Autodesk Fusion 360 part; units mm, degrees
(part 2 of 5)
  spline S130 degree 3 poles (60.3737, -55.5609) (60.3438, -55.5896) (60.2486, -55.657) (60.1179, -55.7383) (59.8305, -55.9172) (59.3718, -56.1632) (59.06, -56.2112) knots 43 43 43 43 44 44 44 45 45 45 45
  spline S131 degree 3 poles (59.06, -56.2112) (58.9588, -56.2268) (58.9104, -56.219) (58.892, -56.2135) knots 45 45 45 45 46 46 46 46
  spline S132 degree 3 poles (58.892, -56.2135) (58.8899, -56.1496) (58.9675, -55.9719) (59.1151, -55.7925) knots 46 46 46 46 47 47 47 47
  ellipse E15 centre (57.3205, -53.9765) end of major axis (56.0356, -51.7283) minor radius 2.1626 (59.1151, -55.7925) -> (59.5802, -54.6452) ccw
  ellipse E16 centre (59.4059, -54.626) end of major axis (59.3998, -54.4501) minor radius 0.1753 (59.5802, -54.6452) -> (59.5256, -54.4974) ccw
  ellipse E17 centre (59.4023, -54.6266) end of major axis (59.2635, -54.7391) minor radius 0.1761 (59.5256, -54.4974) -> (59.3747, -54.4521) ccw
  spline S133 degree 3 poles (59.3747, -54.4521) (55.9933, -55.04) (49.7205, -55.3474) (45.6899, -50.8019) knots 50 50 50 50 51 51 51 51
  ellipse E18 centre (53.6278, -44.8754) end of major axis (44.2457, -38.0609) minor radius 9.7795 (43.9053, -48.2176) -> (45.6899, -50.8019) ccw
  line L25 (43.9053, -48.2176) -> (43.8433, -48.0971)
  ellipse E19 centre (49.3851, -44.1794) end of major axis (52.1384, -53.1388) minor radius 6.6191 (42.9149, -45.6233) -> (43.8433, -48.0971) ccw
  ellipse E20 centre (51.6421, -43.1384) end of major axis (52.985, -53.2351) minor radius 9.0542 (42.8875, -40.1596) -> (42.9149, -45.6233) ccw
  arc A2 (42.8875, -40.1596) -> (42.9826, -39.7986) centre (53.3142, -42.7132) cw
  ellipse E21 centre (42.8151, -39.7494) end of major axis (42.7434, -39.5895) minor radius 0.1739 (42.9826, -39.7986) -> (42.9638, -39.6591) ccw
  spline S134 degree 3 poles (42.9638, -39.6591) (42.3811, -38.6984) (41.6291, -37.8042) (40.8669, -37.0262) (39.8868, -36.026) (38.8897, -35.2179) (38.2132, -34.708) (37.6172, -34.2587) (37.2267, -34.0054) (37.2179, -34.0001) knots 57 57 57 57 58 58 58 59 59 59 60 60 60 60
  ellipse E22 centre (35.2958, -35.3818) end of major axis (31.3426, -33.1165) minor radius 2.2062 (37.2179, -34.0001) -> (36.1564, -33.3367) ccw
  spline S135 degree 3 poles (36.1564, -33.3367) (36.076, -33.2937) (35.9763, -33.3192) (35.9263, -33.3948) knots 61 61 61 61 62 62 62 62
  line L26 (35.9263, -33.3948) -> (35.5901, -33.9003)
  spline S136 degree 3 poles (35.5901, -33.9003) (34.94, -34.8769) (34.2677, -35.8869) (33.6646, -36.9182) knots 63 63 63 63 64 64 64 64
  spline S137 degree 3 poles (33.6646, -36.9182) (33.2824, -37.5723) (32.9384, -38.2578) (32.6058, -38.9206) knots 64 64 64 64 65 65 65 65
  spline S138 degree 3 poles (32.6058, -38.9206) (32.2773, -39.5755) (31.9376, -40.2527) (31.5629, -40.8949) (31.5163, -40.9748) (31.47, -41.0529) (31.4239, -41.1294) knots 65 65 65 65 66 66 66 67 67 67 67
  spline S139 degree 3 poles (31.4239, -41.1294) (31.1015, -41.6648) (30.7918, -42.1186) (30.481, -42.5114) knots 67 67 67 67 68 68 68 68
  line L27 (30.481, -42.5114) -> (30.4362, -42.5696)
  spline S140 degree 3 poles (30.4362, -42.5696) (30.4117, -42.6016) (30.3873, -42.6336) (30.362, -42.6641) knots 69 69 69 69 70 70 70 70
  spline S141 degree 3 poles (30.362, -42.6641) (30.3582, -42.6686) (30.3547, -42.6734) (30.3515, -42.6783) knots 70 70 70 70 71 71 71 71
  spline S142 degree 3 poles (30.3515, -42.6783) (30.3203, -42.7234) (28.6461, -45.1229) (26.2909, -45.4412) knots 71 71 71 71 72 72 72 72
  ellipse E23 centre (26.3128, -35.2005) end of major axis (25.464, -45.4631) minor radius 6.2326 (24.6688, -45.3108) -> (26.2909, -45.4412) ccw
  spline S143 degree 3 poles (24.6688, -45.3108) (24.6431, -45.2963) (24.618, -45.2804) (24.5928, -45.2647) knots 73 73 73 73 74 74 74 74
  line L28 (24.5928, -45.2647) -> (24.5503, -45.2383)
  spline S144 degree 3 poles (24.5503, -45.2383) (24.3504, -45.1156) (24.1596, -44.9484) (23.9667, -44.7273) knots 75 75 75 75 76 76 76 76
  spline S145 degree 3 poles (23.9667, -44.7273) (23.8509, -44.594) (23.7755, -44.4771) (23.7295, -44.3593) knots 76 76 76 76 77 77 77 77
  ellipse E24 centre (23.8379, -44.243) end of major axis (24.0045, -44.7223) minor radius 0.1422 (23.6258, -43.858) -> (23.7295, -44.3593) ccw
  ellipse E25 centre (25.0663, -43.2544) end of major axis (23.7372, -44.3058) minor radius 0.9128 (23.7072, -43.5372) -> (23.6258, -43.858) ccw
  ellipse E26 centre (23.7572, -43.5067) end of major axis (23.6649, -43.7209) minor radius 0.0345 (23.7632, -43.412) -> (23.7072, -43.5372) ccw
  spline S146 degree 3 poles (23.7632, -43.412) (23.9002, -43.2702) (24.0362, -43.1231) (24.1722, -42.9764) knots 80 80 80 80 81 81 81 81
  line L29 (24.1722, -42.9764) -> (24.3262, -42.8105)
  ellipse E27 centre (22.2632, -42.3236) end of major axis (19.1066, -44.8285) minor radius 1.7599 (24.3262, -42.8105) -> (24.9513, -42.0428) ccw
  spline S147 degree 3 poles (24.9513, -42.0428) (25.0276, -41.933) (25.103, -41.8145) (25.1819, -41.6801) knots 83 83 83 83 84 84 84 84
  spline S148 degree 3 poles (25.1819, -41.6801) (25.1991, -41.6508) (25.215, -41.6211) (25.231, -41.5914) knots 84 84 84 84 85 85 85 85
  line L30 (25.231, -41.5914) -> (25.2527, -41.5513)
  spline S149 degree 3 poles (25.2527, -41.5513) (25.2973, -41.4707) (25.3416, -41.3895) (25.3826, -41.3066) knots 86 86 86 86 87 87 87 87
  spline S150 degree 3 poles (25.3826, -41.3066) (25.4022, -41.2663) (25.4208, -41.2258) (25.4396, -41.1853) knots 87 87 87 87 88 88 88 88
  line L31 (25.4396, -41.1853) -> (25.4579, -41.1455)
  spline S151 degree 3 poles (25.4579, -41.1455) (25.4913, -41.0727) (25.5238, -40.9995) (25.5543, -40.9255) (25.5791, -40.8653) (25.6029, -40.8046) (25.626, -40.7437) knots 89 89 89 89 90 90 90 91 91 91 91
  spline S152 degree 3 poles (25.626, -40.7437) (25.6517, -40.6761) (25.6761, -40.6074) (25.6997, -40.5385) knots 91 91 91 91 92 92 92 92
  spline S153 degree 3 poles (25.6997, -40.5385) (25.7223, -40.4724) (25.7448, -40.4057) (25.7657, -40.3384) knots 92 92 92 92 93 93 93 93
  spline S154 degree 3 poles (25.7657, -40.3384) (25.7846, -40.277) (25.802, -40.2143) (25.8187, -40.1532) knots 93 93 93 93 94 94 94 94
  line L32 (25.8187, -40.1532) -> (25.8311, -40.1093)
  spline S155 degree 3 poles (25.8311, -40.1093) (25.848, -40.0494) (25.8649, -39.9896) (25.8804, -39.9277) knots 95 95 95 95 96 96 96 96
  line L33 (25.8804, -39.9277) -> (25.9066, -39.8117)
  spline S156 degree 3 poles (25.9066, -39.8117) (25.9578, -39.5907) (26, -39.3731) (26.0332, -39.1571) (26.1059, -38.6843) (26.1474, -38.1845) (26.1602, -37.6287) knots 97 97 97 97 98 98 98 99 99 99 99
  line L34 (26.1602, -37.6287) -> (26.1614, -37.5503)
  spline S157 degree 3 poles (26.1614, -37.5503) (26.1634, -37.4115) (26.1648, -37.2726) (26.1634, -37.1358) knots 100 100 100 100 101 101 101 101
  line L35 (26.1634, -37.1358) -> (26.1622, -37.0204)
  spline S158 degree 3 poles (26.1622, -37.0204) (26.1607, -36.8934) (26.1581, -36.7667) (26.1539, -36.6415) knots 102 102 102 102 103 103 103 103
  line L36 (26.1539, -36.6415) -> (26.1496, -36.5105)
  spline S159 degree 3 poles (26.1496, -36.5105) (26.145, -36.3889) (26.1397, -36.2682) (26.1333, -36.1463) knots 104 104 104 104 105 105 105 105
  line L37 (26.1333, -36.1463) -> (26.1266, -36.0149)
  spline S160 degree 3 poles (26.1266, -36.0149) (26.1195, -35.8921) (26.1119, -35.7703) (26.1037, -35.6507) knots 106 106 106 106 107 107 107 107
  line L38 (26.1037, -35.6507) -> (26.0961, -35.5324)
  spline S161 degree 3 poles (26.0961, -35.5324) (26.0852, -35.376) (26.0738, -35.2208) (26.0618, -35.0674) (26.0421, -34.8173) (26.0218, -34.5675) (26.0015, -34.3178) (25.98, -34.0538) (25.9584, -33.7898) (25.9378, -33.5252) knots 108 108 108 108 109 109 109 110 110 110 111 111 111 111
  spline S162 degree 3 poles (25.9378, -33.5252) (25.9371, -33.5162) (25.9357, -33.5074) (25.9336, -33.4988) knots 111 111 111 111 112 112 112 112
  line L39 (25.9336, -33.4988) -> (25.9306, -33.464)
  spline S163 degree 3 poles (25.9306, -33.464) (25.9294, -33.4503) (25.9283, -33.4366) (25.927, -33.4216) knots 113 113 113 113 114 114 114 114
  spline S164 degree 3 poles (25.927, -33.4216) (25.925, -33.3993) (25.9229, -33.3745) (25.9208, -33.3495) knots 114 114 114 114 115 115 115 115
  spline S165 degree 3 poles (25.9208, -33.3495) (25.9196, -33.3359) (25.9185, -33.3227) (25.9172, -33.3084) knots 115 115 115 115 116 116 116 116
  spline S166 degree 3 poles (25.9172, -33.3084) (25.9146, -33.2781) (25.9119, -33.2454) (25.909, -33.2118) (25.9081, -33.2012) (25.9073, -33.191) (25.9063, -33.18) knots 116 116 116 116 117 117 117 118 118 118 118
  spline S167 degree 3 poles (25.9063, -33.18) (25.9034, -33.1453) (25.9003, -33.1082) (25.8971, -33.0705) knots 118 118 118 118 119 119 119 119
  spline S168 degree 3 poles (25.8971, -33.0705) (25.896, -33.0568) (25.8949, -33.0437) (25.8937, -33.0296) knots 119 119 119 119 120 120 120 120
  spline S169 degree 3 poles (25.8937, -33.0296) (25.8907, -32.994) (25.8876, -32.9561) (25.8844, -32.9181) knots 120 120 120 120 121 121 121 121
  spline S170 degree 3 poles (25.8844, -32.9181) (25.8827, -32.8984) (25.8812, -32.8793) (25.8795, -32.859) knots 121 121 121 121 122 122 122 122
  spline S171 degree 3 poles (25.8795, -32.859) (25.8768, -32.8266) (25.874, -32.7925) (25.8712, -32.7586) knots 122 122 122 122 123 123 123 123
  line L40 (25.8712, -32.7586) -> (25.8643, -32.6743)
  spline S172 degree 3 poles (25.8643, -32.6743) (25.8616, -32.6416) (25.8589, -32.6075) (25.8561, -32.5735) knots 124 124 124 124 125 125 125 125
  spline S173 degree 3 poles (25.8561, -32.5735) (25.8538, -32.5439) (25.8514, -32.5146) (25.8489, -32.4841) knots 125 125 125 125 126 126 126 126
  spline S174 degree 3 poles (25.8489, -32.4841) (25.8459, -32.4468) (25.8428, -32.408) (25.8398, -32.3695) knots 126 126 126 126 127 127 127 127
  spline S175 degree 3 poles (25.8398, -32.3695) (25.8373, -32.3384) (25.8348, -32.3078) (25.8323, -32.276) knots 127 127 127 127 128 128 128 128
  spline S176 degree 3 poles (25.8323, -32.276) (25.8295, -32.2409) (25.8267, -32.2044) (25.8238, -32.1684) knots 128 128 128 128 129 129 129 129
  spline S177 degree 3 poles (25.8238, -32.1684) (25.8209, -32.1317) (25.8181, -32.0952) (25.8151, -32.0577) knots 129 129 129 129 130 130 130 130
  spline S178 degree 3 poles (25.8151, -32.0577) (25.812, -32.0184) (25.8089, -31.978) (25.8058, -31.9378) knots 130 130 130 130 131 131 131 131
  spline S179 degree 3 poles (25.8058, -31.9378) (25.8032, -31.9041) (25.8006, -31.8707) (25.798, -31.8364) knots 131 131 131 131 132 132 132 132
  spline S180 degree 3 poles (25.798, -31.8364) (25.794, -31.7852) (25.7901, -31.7329) (25.7861, -31.6805) knots 132 132 132 132 133 133 133 133
  spline S181 degree 3 poles (25.7861, -31.6805) (25.7842, -31.656) (25.7824, -31.6318) (25.7805, -31.6069) knots 133 133 133 133 134 134 134 134
  spline S182 degree 3 poles (25.7805, -31.6069) (25.7765, -31.5529) (25.7724, -31.4979) (25.7683, -31.4428) knots 134 134 134 134 135 135 135 135
  spline S183 degree 3 poles (25.7683, -31.4428) (25.7663, -31.4157) (25.7643, -31.3889) (25.7622, -31.3615) knots 135 135 135 135 136 136 136 136
  spline S184 degree 3 poles (25.7622, -31.3615) (25.7584, -31.3084) (25.7544, -31.2545) (25.7505, -31.2006) knots 136 136 136 136 137 137 137 137
  spline S185 degree 3 poles (25.7505, -31.2006) (25.7484, -31.1715) (25.7463, -31.1426) (25.7442, -31.1133) (25.7405, -31.0623) (25.7368, -31.0107) (25.7332, -30.9591) knots 137 137 137 137 138 138 138 139 139 139 139
  spline S186 degree 3 poles (25.7332, -30.9591) (25.7307, -30.9247) (25.7283, -30.8905) (25.7259, -30.8558) knots 139 139 139 139 140 140 140 140
  spline S187 degree 3 poles (25.7259, -30.8558) (25.722, -30.8009) (25.7182, -30.7456) (25.7144, -30.6902) (25.7124, -30.6617) (25.7104, -30.6333) (25.7085, -30.6046) knots 140 140 140 140 141 141 141 142 142 142 142
  spline S188 degree 3 poles (25.7085, -30.6046) (25.7045, -30.5466) (25.7006, -30.4883) (25.6967, -30.4299) knots 142 142 142 142 143 143 143 143
  spline S189 degree 3 poles (25.6967, -30.4299) (25.6948, -30.4007) (25.6928, -30.3716) (25.6908, -30.3424) (25.6869, -30.2824) (25.683, -30.2223) (25.6791, -30.1622) knots 143 143 143 143 144 144 144 145 145 145 145
  spline S190 degree 3 poles (25.6791, -30.1622) (25.6775, -30.136) (25.6758, -30.11) (25.6741, -30.0838) knots 145 145 145 145 146 146 146 146
  spline S191 degree 3 poles (25.6741, -30.0838) (25.6703, -30.0249) (25.6667, -29.966) (25.663, -29.9072) knots 146 146 146 146 147 147 147 147
  spline S192 degree 3 poles (25.663, -29.9072) (25.6613, -29.878) (25.6594, -29.8489) (25.6576, -29.8198) knots 147 147 147 147 148 148 148 148
  spline S193 degree 3 poles (25.6576, -29.8198) (25.6543, -29.766) (25.6512, -29.7126) (25.648, -29.659) knots 148 148 148 148 149 149 149 149
  spline S194 degree 3 poles (25.648, -29.659) (25.646, -29.6254) (25.644, -29.5917) (25.642, -29.5582) knots 149 149 149 149 150 150 150 150
  spline S195 degree 3 poles (25.642, -29.5582) (25.6391, -29.5083) (25.6364, -29.4588) (25.6336, -29.4093) (25.6315, -29.3726) (25.6294, -29.3357) (25.6274, -29.2992) knots 150 150 150 150 151 151 151 152 152 152 152
  spline S196 degree 3 poles (25.6274, -29.2992) (25.6247, -29.2508) (25.6222, -29.203) (25.6197, -29.1549) knots 152 152 152 152 153 153 153 153
  spline S197 degree 3 poles (25.6197, -29.1549) (25.6178, -29.1185) (25.6158, -29.0819) (25.6139, -29.0458) (25.6113, -28.9946) (25.6088, -28.9443) (25.6064, -28.8937) knots 153 153 153 153 154 154 154 155 155 155 155
  spline S198 degree 3 poles (25.6064, -28.8937) (25.6048, -28.8617) (25.6032, -28.8292) (25.6017, -28.7975) knots 155 155 155 155 156 156 156 156
  spline S199 degree 3 poles (25.6017, -28.7975) (25.5994, -28.7483) (25.5972, -28.7001) (25.5951, -28.6517) (25.5936, -28.6187) (25.5921, -28.5851) (25.5906, -28.5525) knots 156 156 156 156 157 157 157 158 158 158 158
  spline S200 degree 3 poles (25.5906, -28.5525) (25.5885, -28.5027) (25.5866, -28.4541) (25.5847, -28.4052) knots 158 158 158 158 159 159 159 159
  spline S201 degree 3 poles (25.5847, -28.4052) (25.5836, -28.3761) (25.5823, -28.3465) (25.5812, -28.3178) (25.5793, -28.2659) (25.5776, -28.2155) (25.5759, -28.1649) knots 159 159 159 159 160 160 160 161 161 161 161
  spline S202 degree 3 poles (25.5759, -28.1649) (25.5751, -28.14) (25.5741, -28.1143) (25.5734, -28.0897) (25.5718, -28.0405) (25.5706, -27.9931) (25.5693, -27.9454) knots 161 161 161 161 162 162 162 163 163 163 163
  spline S203 degree 3 poles (25.5693, -27.9454) (25.5687, -27.9206) (25.5679, -27.895) (25.5672, -27.8706) knots 163 163 163 163 164 164 164 164
  spline S204 degree 3 poles (25.5672, -27.8706) (25.5662, -27.8283) (25.5655, -27.7878) (25.5648, -27.7468) knots 164 164 164 164 165 165 165 165
  spline S205 degree 3 poles (25.5648, -27.7468) (25.5642, -27.7186) (25.5635, -27.6894) (25.563, -27.6618) (25.5623, -27.6174) (25.562, -27.5752) (25.5616, -27.5326) knots 165 165 165 165 166 166 166 167 167 167 167
  spline S206 degree 3 poles (25.5616, -27.5326) (25.5614, -27.511) (25.561, -27.4884) (25.5609, -27.4673) knots 167 167 167 167 168 168 168 168
  spline S207 degree 3 poles (25.5609, -27.4673) (25.5607, -27.4265) (25.5608, -27.388) (25.5609, -27.349) knots 168 168 168 168 169 169 169 169
  spline S208 degree 3 poles (25.5609, -27.349) (25.561, -27.3275) (25.5608, -27.3047) (25.561, -27.2838) knots 169 169 169 169 170 170 170 170
  spline S209 degree 3 poles (25.561, -27.2838) (25.5612, -27.2469) (25.5619, -27.2126) (25.5624, -27.1777) knots 170 170 170 170 171 171 171 171
  spline S210 degree 3 poles (25.5624, -27.1777) (25.5628, -27.1573) (25.5629, -27.1355) (25.5633, -27.1158) knots 171 171 171 171 172 172 172 172
  spline S211 degree 3 poles (25.5633, -27.1158) (25.5642, -27.0762) (25.5655, -27.0395) (25.5669, -27.0029) knots 172 172 172 172 173 173 173 173
  spline S212 degree 3 poles (25.5669, -27.0029) (25.5673, -26.99) (25.5676, -26.9758) (25.5681, -26.9633) knots 173 173 173 173 174 174 174 174
  spline S213 degree 3 poles (25.5681, -26.9633) (25.5701, -26.9151) (25.5726, -26.8697) (25.5755, -26.8274) (25.5894, -26.6266) (25.6138, -26.3766) (25.6465, -26.0916) (25.8752, -24.0967) (26.5072, -20.3884) (26.7336, -19.8514) knots 174 174 174 174 175 175 175 176 176 176 177 177 177 177
  spline S214 degree 3 poles (72.9313, -24.8062) (72.9855, -24.4014) (73.0419, -23.9826) (73.0388, -23.5465) knots 0 0 0 0 1 1 1 1
  line L41 (73.0388, -23.5465) -> (73.0374, -23.4045)
  spline S215 degree 3 poles (73.0374, -23.4045) (73.0357, -23.2452) (73.0339, -23.0803) (73.0403, -22.9205) knots 2 2 2 2 3 3 3 3
  spline S216 degree 3 poles (73.0403, -22.9205) (73.0434, -22.8442) (73.0427, -22.7594) (73.0417, -22.6709) knots 3 3 3 3 4 4 4 4
  spline S217 degree 3 poles (73.0417, -22.6709) (73.0409, -22.597) (73.0401, -22.5187) (73.0421, -22.4407) knots 4 4 4 4 5 5 5 5
  spline S218 degree 3 poles (73.0421, -22.4407) (73.0421, -22.4393) (73.0422, -22.4379) (73.0423, -22.4366) knots 5 5 5 5 6 6 6 6
  spline S219 degree 3 poles (73.0423, -22.4366) (73.0485, -22.2022) (73.0805, -21.9711) (73.2153, -21.8725) knots 6 6 6 6 7 7 7 7
  spline S220 degree 3 poles (73.2153, -21.8725) (73.216, -21.872) (73.2168, -21.8715) (73.2176, -21.871) knots 7 7 7 7 8 8 8 8
  spline S221 degree 3 poles (73.2176, -21.871) (73.2256, -21.8651) (73.2342, -21.8604) (73.2424, -21.8548) knots 8 8 8 8 9 9 9 9
  line L42 (73.2424, -21.8548) -> (73.2617, -21.8427)
  spline S222 degree 3 poles (73.2617, -21.8427) (73.2624, -21.8422) (73.2629, -21.8415) (73.2636, -21.841) knots 10 10 10 10 11 11 11 11
  spline S223 degree 3 poles (73.2636, -21.841) (73.3094, -21.8113) (73.3567, -21.7841) (73.4081, -21.7615) knots 11 11 11 11 12 12 12 12
  spline S224 degree 3 poles (73.4081, -21.7615) (74.0725, -21.4735) (74.8812, -21.7752) (75.5947, -22.0411) knots 12 12 12 12 13 13 13 13
  spline S225 degree 3 poles (75.5947, -22.0411) (75.6925, -22.0776) (75.788, -22.1131) (75.8805, -22.1462) knots 13 13 13 13 14 14 14 14
  spline S226 degree 3 poles (75.8805, -22.1462) (76.5283, -22.3777) (77.3298, -22.7517) (77.782, -23.5961) knots 14 14 14 14 15 15 15 15
  ellipse E28 centre (73.2621, -23.0014) end of major axis (68.6988, -22.1892) minor radius 1.1094 (77.7908, -23.9063) -> (77.782, -23.5961) ccw
  spline S227 degree 3 poles (77.7908, -23.9063) (77.7219, -24.0239) (77.5651, -24.1149) (77.4261, -24.1176) knots 16 16 16 16 17 17 17 17
  spline S228 degree 3 poles (77.4261, -24.1176) (77.422, -24.1178) (77.4177, -24.1178) (77.4135, -24.1178) (77.2368, -24.1178) (77.0589, -24.0482) (76.8706, -23.9745) knots 17 17 17 17 18 18 18 19 19 19 19
  spline S229 degree 3 poles (76.8706, -23.9745) (76.7481, -23.9266) (76.6215, -23.8772) (76.4889, -23.8448) knots 19 19 19 19 20 20 20 20
  spline S230 degree 3 poles (76.4889, -23.8448) (76.0338, -23.734) (75.4354, -23.6331) (74.8433, -23.8376) knots 20 20 20 20 21 21 21 21
  spline S231 degree 3 poles (74.8433, -23.8376) (74.5553, -23.937) (74.411, -24.0675) (74.4018, -24.237) knots 21 21 21 21 22 22 22 22
  spline S232 degree 3 poles (74.4018, -24.237) (74.3892, -24.4694) (74.6475, -24.5907) (74.7322, -24.6305) knots 22 22 22 22 23 23 23 23
  spline S233 degree 3 poles (74.7322, -24.6305) (75.208, -24.8546) (75.7108, -24.8582) (76.1971, -24.8618) knots 23 23 23 23 24 24 24 24
  spline S234 degree 3 poles (76.1971, -24.8618) (76.2789, -24.8625) (76.3604, -24.863) (76.4413, -24.8647) knots 24 24 24 24 25 25 25 25
  spline S235 degree 3 poles (76.4413, -24.8647) (76.4902, -24.8658) (76.5416, -24.8661) (76.5945, -24.8664) knots 25 25 25 25 26 26 26 26
  spline S236 degree 3 poles (76.5945, -24.8664) (76.9596, -24.869) (77.414, -24.8723) (77.6507, -25.1272) knots 26 26 26 26 27 27 27 27
  spline S237 degree 3 poles (77.6507, -25.1272) (77.788, -25.2757) (77.819, -25.5634) (77.655, -25.7262) knots 27 27 27 27 28 28 28 28
  ellipse E29 centre (76.3477, -25.5008) end of major axis (74.4768, -26.6804) minor radius 0.9918 (76.3888, -26.6097) -> (77.655, -25.7262) ccw
  spline S238 degree 3 poles (76.3888, -26.6097) (75.639, -26.969) (74.6962, -27.1357) (73.8024, -27.0653) knots 29 29 29 29 30 30 30 30
  line L43 (73.8024, -27.0653) -> (73.8022, -27.0653)
  spline S239 degree 3 poles (73.8022, -27.0653) (73.5657, -27.0469) (73.3311, -27.0114) (73.1471, -26.9108) knots 31 31 31 31 32 32 32 32
  spline S240 degree 3 poles (73.1471, -26.9108) (73.1453, -26.9097) (73.1441, -26.908) (73.1423, -26.907) knots 32 32 32 32 33 33 33 33
  spline S241 degree 3 poles (73.1423, -26.907) (73.0965, -26.8817) (73.0567, -26.8539) (73.0212, -26.8235) knots 33 33 33 33 34 34 34 34
  spline S242 degree 3 poles (73.0212, -26.8235) (73.0189, -26.8215) (73.0164, -26.8198) (73.0142, -26.8178) knots 34 34 34 34 35 35 35 35
  spline S243 degree 3 poles (73.0142, -26.8178) (72.9786, -26.7865) (72.9478, -26.7525) (72.9218, -26.7149) knots 35 35 35 35 36 36 36 36
  spline S244 degree 3 poles (72.9218, -26.7149) (72.7787, -26.5077) (72.7974, -26.2505) (72.8193, -25.9529) knots 36 36 36 36 37 37 37 37
  spline S245 degree 3 poles (72.8193, -25.9529) (72.8241, -25.887) (72.829, -25.8211) (72.8321, -25.7553) knots 37 37 37 37 38 38 38 38
  spline S246 degree 3 poles (72.8321, -25.7553) (72.8467, -25.4354) (72.8898, -25.1155) (72.9313, -24.8062) knots 38 38 38 38 39 39 39 39
  spline S247 degree 3 poles (39.324, -44.6943) (38.6743, -45.7946) (38.1289, -46.8331) (37.657, -47.8689) knots 0 0 0 0 1 1 1 1
  spline S248 degree 3 poles (37.657, -47.8689) (37.5615, -48.0777) (37.462, -48.2878) (37.3612, -48.4994) knots 1 1 1 1 2 2 2 2
  ellipse E30 centre (56.5312, -70.3059) end of major axis (34.791, -46.1267) minor radius 0.7215 (37.3612, -48.4994) -> (35.471, -46.6399) ccw
  ellipse E31 centre (35.3066, -46.7125) end of major axis (35.1243, -46.693) minor radius 0.1699 (35.471, -46.6399) -> (35.4278, -46.5867) ccw
  spline S249 degree 3 poles (35.4278, -46.5867) (34.7297, -46.0091) (34.0382, -45.4165) (33.436, -44.8979) knots 4 4 4 4 5 5 5 5
  spline S250 degree 3 poles (33.436, -44.8979) (34.7307, -41.3001) (36.7571, -37.4286) (38.1563, -35.1078) knots 5 5 5 5 6 6 6 6
  spline S251 degree 3 poles (38.1563, -35.1078) (39.3533, -36.0256) (41.3728, -37.7507) (42.6224, -39.7771) knots 6 6 6 6 7 7 7 7
  spline S252 degree 3 poles (42.6224, -39.7771) (42.5984, -39.8641) (42.5755, -39.9514) (42.5538, -40.039) knots 7 7 7 7 8 8 8 8
  spline S253 degree 3 poles (42.5538, -40.039) (41.1796, -41.8118) (40.1529, -43.2918) (39.324, -44.6943) knots 8 8 8 8 9 9 9 9
  spline S254 degree 3 poles (30.8632, -42.5945) (30.8664, -42.5904) (30.8695, -42.5858) (30.8727, -42.5817) knots 0 0 0 0 1 1 1 1
  spline S255 degree 3 poles (30.8727, -42.5817) (30.9459, -42.4856) (31.0192, -42.3857) (31.0926, -42.2826) knots 1 1 1 1 2 2 2 2
  spline S256 degree 3 poles (31.0926, -42.2826) (31.1038, -42.2669) (31.115, -42.2512) (31.1263, -42.2352) knots 2 2 2 2 3 3 3 3
  spline S257 degree 3 poles (31.1263, -42.2352) (31.199, -42.1321) (31.272, -42.0252) (31.3453, -41.9146) knots 3 3 3 3 4 4 4 4
  spline S258 degree 3 poles (31.3453, -41.9146) (31.3565, -41.8978) (31.3677, -41.8806) (31.3789, -41.8635) knots 4 4 4 4 5 5 5 5
  spline S259 degree 3 poles (31.3789, -41.8635) (31.4533, -41.7502) (31.528, -41.6334) (31.6034, -41.5119) knots 5 5 5 5 6 6 6 6
  spline S260 degree 3 poles (31.6034, -41.5119) (31.6118, -41.4984) (31.6202, -41.4843) (31.6286, -41.4707) knots 6 6 6 6 7 7 7 7
  spline S261 degree 3 poles (31.6286, -41.4707) (31.7076, -41.3424) (31.787, -41.2106) (31.8675, -41.0727) knots 7 7 7 7 8 8 8 8
  line L44 (31.8675, -41.0727) -> (31.8676, -41.0727)
  spline S262 degree 3 poles (31.8676, -41.0727) (32.1528, -40.5838) (32.4166, -40.0778) (32.6703, -39.577) knots 9 9 9 9 10 10 10 10
  spline S263 degree 3 poles (32.6703, -39.577) (32.7549, -39.4101) (32.8384, -39.2438) (32.9212, -39.0788) knots 10 10 10 10 11 11 11 11
  spline S264 degree 3 poles (32.9212, -39.0788) (33.2512, -38.4209) (33.5926, -37.7405) (33.9691, -37.0962) knots 11 11 11 11 12 12 12 12
  spline S265 degree 3 poles (33.9691, -37.0962) (34.5669, -36.0739) (35.2364, -35.0682) (35.8838, -34.0958) knots 12 12 12 12 13 13 13 13
  line L45 (35.8838, -34.0958) -> (36.1306, -33.7246)
  ellipse E32 centre (30.0181, -45.084) end of major axis (24.3221, -56.662) minor radius 10.7769 (37.0187, -34.2911) -> (36.1306, -33.7246) ccw
  spline S266 degree 3 poles (37.0187, -34.2911) (37.0195, -34.2916) (37.0376, -34.3035) (37.0653, -34.3218) knots 15 15 15 15 16 16 16 16
  spline S267 degree 3 poles (37.0653, -34.3218) (37.0718, -34.3262) (37.0768, -34.3294) (37.0847, -34.3347) knots 16 16 16 16 17 17 17 17
  spline S268 degree 3 poles (37.0847, -34.3347) (37.0933, -34.3405) (37.1056, -34.3488) (37.1158, -34.3557) knots 17 17 17 17 18 18 18 18
  spline S269 degree 3 poles (37.1158, -34.3557) (37.1313, -34.3661) (37.1472, -34.3768) (37.1662, -34.3898) knots 18 18 18 18 19 19 19 19
  spline S270 degree 3 poles (37.1662, -34.3898) (37.1775, -34.3974) (37.1911, -34.4068) (37.2035, -34.4153) knots 19 19 19 19 20 20 20 20
  spline S271 degree 3 poles (37.2035, -34.4153) (37.2258, -34.4305) (37.2492, -34.4466) (37.2752, -34.4646) knots 20 20 20 20 21 21 21 21
  spline S272 degree 3 poles (37.2752, -34.4646) (37.2903, -34.475) (37.3071, -34.4868) (37.3233, -34.498) knots 21 21 21 21 22 22 22 22
  spline S273 degree 3 poles (37.3233, -34.498) (37.3502, -34.5167) (37.3783, -34.5364) (37.4082, -34.5575) knots 22 22 22 22 23 23 23 23
  spline S274 degree 3 poles (37.4082, -34.5575) (37.4277, -34.5712) (37.4484, -34.5859) (37.4691, -34.6006) knots 23 23 23 23 24 24 24 24
  ellipse E33 centre (39.3547, -36.1342) end of major axis (37.0349, -34.3267) minor radius 0.0902 (37.565, -34.6691) -> (37.4691, -34.6006) ccw
  ellipse E34 centre (37.7072, -34.7796) end of major axis (37.3609, -34.5272) minor radius 0.0062 (37.6386, -34.7222) -> (37.565, -34.6691) ccw
  spline S275 degree 3 poles (37.6386, -34.7222) (37.6722, -34.7465) (37.7071, -34.772) (37.7427, -34.7981) knots 26 26 26 26 27 27 27 27
  spline S276 degree 3 poles (37.7427, -34.7981) (37.7704, -34.8183) (37.7985, -34.839) (37.8273, -34.8603) knots 27 27 27 27 28 28 28 28
  spline S277 degree 3 poles (37.8273, -34.8603) (37.8421, -34.8713) (37.858, -34.8832) (37.8731, -34.8945) knots 28 28 28 28 29 29 29 29
  spline S278 degree 3 poles (37.8731, -34.8945) (37.8684, -34.9023) (37.8633, -34.911) (37.8586, -34.9189) knots 29 29 29 29 30 30 30 30
  ellipse E35 centre (32.6135, -46.6373) end of major axis (39.2145, -33.1163) minor radius 0.8189 (37.8586, -34.9189) -> (37.6192, -35.3205) ccw
  spline S279 degree 3 poles (37.6192, -35.3205) (37.6103, -35.3358) (37.6014, -35.3509) (37.5924, -35.3663) knots 31 31 31 31 32 32 32 32
  ellipse E36 centre (-9.0792, -151.5856) end of major axis (39.8086, -32.5747) minor radius 4.3167 (37.5924, -35.3663) -> (37.3338, -35.8113) ccw
  line L46 (37.3338, -35.8113) -> (37.3141, -35.8456)
  arc A3 (37.3141, -35.8456) -> (37.0376, -36.3335) centre (86.78, -64.2077) ccw
  spline S280 degree 3 poles (37.0376, -36.3335) (37.0338, -36.3402) (37.0301, -36.347) (37.0263, -36.3537) knots 35 35 35 35 36 36 36 36
  arc A4 (37.0263, -36.3537) -> (36.7324, -36.8846) centre (91.0882, -66.6257) ccw
  line L47 (36.7324, -36.8846) -> (36.7316, -36.886)
  ellipse E37 centre (37.1187, -39.0776) end of major axis (41.5085, -30.5194) minor radius 1.3681 (36.7316, -36.886) -> (34.8533, -40.5897) ccw
  spline S281 degree 3 poles (34.8533, -40.5897) (34.8532, -40.5898) (34.8532, -40.59) (34.8532, -40.5901) knots 39 39 39 39 40 40 40 40
  ellipse E38 centre (34.2101, -54.8401) end of major axis (40.4764, -33.4497) minor radius 4.3266 (34.8532, -40.5901) -> (34.5529, -41.2419) ccw
  spline S282 degree 3 poles (34.5529, -41.2419) (34.5491, -41.2503) (34.5453, -41.2586) (34.5415, -41.267) knots 41 41 41 41 42 42 42 42
  spline S283 degree 3 poles (34.5415, -41.267) (34.4453, -41.4791) (34.3504, -41.6924) (34.2566, -41.9063) knots 42 42 42 42 43 43 43 43
  spline S284 degree 3 poles (34.2566, -41.9063) (34.2501, -41.9213) (34.2436, -41.9361) (34.237, -41.951) knots 43 43 43 43 44 44 44 44
  arc A5 (34.237, -41.951) -> (33.9665, -42.5807) centre (82.7186, -63.15) ccw
  spline S285 degree 3 poles (33.9665, -42.5807) (33.9584, -42.5999) (33.9503, -42.619) (33.9423, -42.6383) knots 45 45 45 45 46 46 46 46
  arc A6 (33.9423, -42.6383) -> (33.686, -43.2596) centre (78.6674, -61.452) ccw
  spline S286 degree 3 poles (33.686, -43.2596) (33.6769, -43.282) (33.6679, -43.3044) (33.6588, -43.3269) knots 47 47 47 47 48 48 48 48
  ellipse E39 centre (48.4895, -33.6508) end of major axis (63.9881, -11.9775) minor radius 8.195 (33.6588, -43.3269) -> (33.4162, -43.9424) ccw
  spline S287 degree 3 poles (33.4162, -43.9424) (33.4073, -43.9655) (33.3986, -43.9885) (33.3897, -44.0116) knots 49 49 49 49 50 50 50 50
  spline S288 degree 3 poles (33.3897, -44.0116) (33.3111, -44.2165) (33.2344, -44.421) (33.1601, -44.6247) knots 50 50 50 50 51 51 51 51
  spline S289 degree 3 poles (33.1601, -44.6247) (33.1569, -44.6336) (33.1533, -44.6426) (33.1501, -44.6515) knots 51 51 51 51 52 52 52 52
  line L48 (33.1501, -44.6515) -> (32.2642, -43.8893)
  spline S290 degree 3 poles (32.2642, -43.8893) (31.786, -43.4123) (31.3264, -42.9875) (30.8632, -42.5945) knots 53 53 53 53 54 54 54 54
  line L49 (38.9947, -50.6983) -> (39.4139, -51.1607)
  spline S291 degree 3 poles (39.4139, -51.1607) (39.9939, -51.8006) (40.5936, -52.4623) (41.1923, -53.106) knots 1 1 1 1 2 2 2 2
  spline S292 degree 3 poles (41.1923, -53.106) (41.2109, -53.126) (41.2299, -53.1454) (41.249, -53.1648) knots 2 2 2 2 3 3 3 3
  line L50 (41.249, -53.1648) -> (41.2958, -53.2134)
  spline S293 degree 3 poles (41.2958, -53.2134) (42.1082, -54.079) (42.9698, -54.9126) (43.8032, -55.7188) knots 4 4 4 4 5 5 5 5
  spline S294 degree 3 poles (43.8032, -55.7188) (44.1279, -56.0328) (44.4526, -56.3469) (44.7756, -56.6639) knots 5 5 5 5 6 6 6 6
  line L51 (44.7756, -56.6639) -> (44.9216, -56.8064)
  spline S295 degree 3 poles (44.9216, -56.8064) (45.0103, -56.8929) (45.099, -56.9793) (45.1869, -57.0668) knots 7 7 7 7 8 8 8 8
  spline S296 degree 3 poles (45.1869, -57.0668) (45.7405, -57.6188) (46.2893, -58.1972) (46.82, -58.7565) knots 8 8 8 8 9 9 9 9
  spline S297 degree 3 poles (46.82, -58.7565) (47.3924, -59.3596) (47.9843, -59.9832) (48.5857, -60.5778) knots 9 9 9 9 10 10 10 10
  arc A7 (48.5857, -60.5778) -> (48.6139, -60.6004) centre (48.7082, -60.4539) ccw
  spline S298 degree 3 poles (48.6139, -60.6004) (49.0142, -60.8595) (49.4054, -61.1682) (49.7837, -61.4667) (50.1992, -61.7946) (50.6289, -62.1337) (51.0725, -62.4082) (52.3821, -63.2189) (53.887, -63.8064) (55.9518, -64.313) (56.5156, -64.4513) (57.1093, -64.574) (57.6835, -64.6926) (59.359, -65.0388) (61.0895, -65.3977) (62.5497, -66.2155) knots 11 11 11 11 12 12 12 13 13 13 14 14 14 15 15 15 16 16 16 16
  spline S299 degree 3 poles (62.5497, -66.2155) (62.5488, -66.4378) (62.5521, -66.6639) (62.5638, -66.8979) knots 16 16 16 16 17 17 17 17
  spline S300 degree 3 poles (62.5638, -66.8979) (62.5677, -66.9776) (62.6248, -67.0446) (62.7026, -67.0615) (62.7591, -67.0737) (63.2455, -67.1755) (63.9532, -67.2278) knots 17 17 17 17 18 18 18 19 19 19 19
  ellipse E40 centre (63.1148, -67.3366) end of major axis (61.9899, -66.7228) minor radius 0.5877 (64.1029, -67.3973) -> (63.9532, -67.2278) ccw
  spline S301 degree 3 poles (64.1029, -67.3973) (64.0388, -67.3899) (63.9774, -67.3806) (63.9127, -67.3737) knots 20 20 20 20 21 21 21 21
  spline S302 degree 3 poles (63.9127, -67.3737) (63.9063, -67.373) (63.9001, -67.3726) (63.8939, -67.3726) (63.8361, -67.3726) (63.7815, -67.4011) (63.7484, -67.4495) knots 21 21 21 21 22 22 22 23 23 23 23
  spline S303 degree 3 poles (63.7484, -67.4495) (63.7317, -67.4739) (63.6389, -67.6127) (63.5123, -67.8428) knots 23 23 23 23 24 24 24 24
  spline S304 degree 3 poles (63.5123, -67.8428) (63.3319, -67.7277) (63.1572, -67.6023) (62.9974, -67.4836) knots 24 24 24 24 25 25 25 25
  spline S305 degree 3 poles (62.9974, -67.4836) (61.2812, -66.438) (59.2241, -66.1928) (57.2347, -65.9557) (56.7376, -65.8964) (56.2234, -65.8351) (55.7342, -65.7625) (54.5012, -65.5795) (53.0596, -65.3198) (51.7172, -64.7813) knots 25 25 25 25 26 26 26 27 27 27 28 28 28 28
  spline S306 degree 3 poles (51.7172, -64.7813) (51.6499, -64.7542) (51.5727, -64.7714) (51.5229, -64.8243) knots 28 28 28 28 29 29 29 29
  spline S307 degree 3 poles (51.5229, -64.8243) (51.4733, -64.8773) (51.4611, -64.9553) (51.4925, -65.0209) knots 29 29 29 29 30 30 30 30
  ellipse E41 centre (35.7984, -66.6089) end of major axis (20.7771, -52.7733) minor radius 13.7431 (53.0616, -69.4946) -> (51.4925, -65.0209) ccw
  spline S308 degree 3 poles (53.0616, -69.4946) (53.0204, -69.5064) (52.9798, -69.5168) (52.9384, -69.529) knots 31 31 31 31 32 32 32 32
  spline S309 degree 3 poles (52.9384, -69.529) (52.8469, -69.556) (52.7935, -69.6507) (52.8178, -69.7429) knots 32 32 32 32 33 33 33 33
  spline S310 degree 3 poles (52.8178, -69.7429) (52.8354, -69.8103) (53.0067, -70.4469) (53.3634, -71.2648) knots 33 33 33 33 34 34 34 34
  ellipse E42 centre (44.4714, -74.3946) end of major axis (42.1725, -86.2454) minor radius 8.8523 (53.4416, -72.223) -> (53.3634, -71.2648) ccw
  spline S311 degree 3 poles (53.4416, -72.223) (53.3894, -72.1315) (53.3548, -72.0742) (53.3437, -72.0559) (53.3149, -72.0087) (53.2656, -71.9777) (53.2105, -71.9722) knots 35 35 35 35 36 36 36 37 37 37 37
  spline S312 degree 3 poles (53.2105, -71.9722) (53.2047, -71.9716) (53.199, -71.9713) (53.1931, -71.9713) (53.1442, -71.9713) (53.097, -71.9917) (53.0636, -72.0281) knots 37 37 37 37 38 38 38 39 39 39 39
  spline S313 degree 3 poles (53.0636, -72.0281) (52.9643, -72.1357) (52.867, -72.2427) (52.771, -72.3493) knots 39 39 39 39 40 40 40 40
  ellipse E43 centre (34.1997, -71.7957) end of major axis (16.7983, -60.5355) minor radius 14.9929 (52.771, -72.3493) -> (51.6621, -69.4691) ccw
  spline S314 degree 3 poles (51.6621, -69.4691) (51.5173, -69.2279) (51.3853, -68.9708) (51.2578, -68.7222) knots 41 41 41 41 42 42 42 42
  spline S315 degree 3 poles (51.2578, -68.7222) (51.186, -68.5822) (51.1135, -68.4426) (51.0389, -68.3039) knots 42 42 42 42 43 43 43 43
  spline S316 degree 3 poles (51.0389, -68.3039) (51.0627, -67.9892) (51.0747, -67.6622) (51.0732, -67.3215) knots 43 43 43 43 44 44 44 44
  spline S317 degree 3 poles (51.0732, -67.3215) (51.0728, -67.2418) (51.0191, -67.1722) (50.9421, -67.1518) knots 44 44 44 44 45 45 45 45
  spline S318 degree 3 poles (50.9421, -67.1518) (50.8992, -67.1404) (50.6077, -67.065) (50.1572, -66.9924) knots 45 45 45 45 46 46 46 46
  line L52 (50.1572, -66.9924) -> (50.0161, -66.8131)
  spline S319 degree 3 poles (50.0161, -66.8131) (49.9403, -66.7172) (49.8646, -66.6214) (49.7897, -66.5253) knots 47 47 47 47 48 48 48 48
  spline S320 degree 3 poles (49.7897, -66.5253) (49.6504, -66.3459) (49.517, -66.1544) (49.388, -65.969) (49.2359, -65.7505) (49.0786, -65.5245) (48.9069, -65.3114) knots 48 48 48 48 49 49 49 50 50 50 50
  spline S321 degree 3 poles (48.9069, -65.3114) (48.3798, -64.6568) (47.7742, -64.0635) (47.1883, -63.4898) knots 50 50 50 50 51 51 51 51
  spline S322 degree 3 poles (47.1883, -63.4898) (47.0202, -63.325) (46.8519, -63.1602) (46.6778, -62.9868) knots 51 51 51 51 52 52 52 52
  line L53 (46.6778, -62.9868) -> (45.39, -61.8458)
  spline S323 degree 3 poles (45.39, -61.8458) (44.4669, -61.0281) (43.5438, -60.2105) (42.6219, -59.3914) knots 53 53 53 53 54 54 54 54
  spline S324 degree 3 poles (42.6219, -59.3914) (42.2253, -59.0389) (41.8279, -58.6871) (41.4307, -58.3353) (39.8976, -56.9774) (38.3145, -55.5743) (36.7915, -54.1534) knots 54 54 54 54 55 55 55 56 56 56 56
  spline S325 degree 3 poles (36.7915, -54.1534) (36.8575, -54.0679) (36.9176, -53.978) (36.9726, -53.8887) knots 56 56 56 56 57 57 57 57
  spline S326 degree 3 poles (36.9726, -53.8887) (37.4349, -53.1365) (37.7121, -52.2325) (37.7334, -51.4085) knots 57 57 57 57 58 58 58 58
  ellipse E44 centre (36.7327, -50.92) end of major axis (36.5209, -48.7344) minor radius 0.9842 (37.7334, -51.4085) -> (37.5238, -49.8874) ccw
  spline S327 degree 3 poles (37.5238, -49.8874) (37.4079, -49.5262) (36.9917, -49.3114) (36.6164, -49.4176) knots 59 59 59 59 60 60 60 60
  spline S328 degree 3 poles (36.6164, -49.4176) (36.1669, -49.5443) (35.9268, -50.006) (35.7515, -50.3432) knots 60 60 60 60 61 61 61 61
  spline S329 degree 3 poles (35.7515, -50.3432) (35.7296, -50.3853) (35.7084, -50.4259) (35.6877, -50.4644) knots 61 61 61 61 62 62 62 62
  spline S330 degree 3 poles (35.6877, -50.4644) (35.6505, -50.5333) (35.6142, -50.6029) (35.5777, -50.6728) knots 62 62 62 62 63 63 63 63
  spline S331 degree 3 poles (35.5777, -50.6728) (35.3797, -51.0522) (35.1927, -51.4106) (34.87, -51.6604) knots 63 63 63 63 64 64 64 64
  ellipse E45 centre (35.0453, -51.3467) end of major axis (34.7131, -51.728) minor radius 0.1029 (34.8001, -51.7086) -> (34.87, -51.6604) ccw
  ellipse E46 centre (35.0937, -51.1581) end of major axis (34.8485, -51.8215) minor radius 0.174 (34.8091, -51.5521) -> (34.8001, -51.7086) ccw
  spline S332 degree 3 poles (34.8091, -51.5521) (34.8625, -51.1738) (35.0528, -50.8122) (35.4259, -50.3798) knots 66 66 66 66 67 67 67 67
  spline S333 degree 3 poles (35.4259, -50.3798) (35.4931, -50.302) (35.5742, -50.2301) (35.6602, -50.154) (35.8214, -50.0112) (35.9881, -49.8635) (36.0908, -49.6527) knots 67 67 67 67 68 68 68 69 69 69 69
  spline S334 degree 3 poles (36.0908, -49.6527) (36.1974, -49.4332) (36.1812, -49.1377) (36.051, -48.9341) knots 69 69 69 69 70 70 70 70
  spline S335 degree 3 poles (36.051, -48.9341) (35.9358, -48.7536) (35.7465, -48.6549) (35.5169, -48.6549) (35.5117, -48.6549) (35.5065, -48.6549) (35.5014, -48.655) knots 70 70 70 70 71 71 71 72 72 72 72
  spline S336 degree 3 poles (35.5014, -48.655) (34.5037, -48.6743) (33.7952, -49.2227) (33.2893, -49.6983) knots 72 72 72 72 73 73 73 73
  spline S337 degree 3 poles (33.2893, -49.6983) (33.224, -49.7598) (33.1554, -49.8226) (33.0851, -49.887) knots 73 73 73 73 74 74 74 74
  spline S338 degree 3 poles (33.0851, -49.887) (32.9423, -50.0179) (32.7903, -50.1576) (32.643, -50.3068) knots 74 74 74 74 75 75 75 75
  spline S339 degree 3 poles (32.643, -50.3068) (31.7466, -49.4832) (30.968, -48.7694) (30.7819, -48.5988) knots 75 75 75 75 76 76 76 76
  line L54 (30.7819, -48.5988) -> (30.7461, -48.566)
  spline S340 degree 3 poles (30.7461, -48.566) (30.7407, -48.5605) (30.7351, -48.5554) (30.729, -48.5507) knots 77 77 77 77 78 78 78 78
  line L55 (30.729, -48.5507) -> (29.7117, -47.7449)
  spline S341 degree 3 poles (29.7117, -47.7449) (29.7077, -47.7413) (29.7034, -47.7378) (29.699, -47.7346) knots 79 79 79 79 80 80 80 80
  spline S342 degree 3 poles (29.699, -47.7346) (29.5143, -47.5979) (29.3339, -47.4674) (29.1627, -47.3434) knots 80 80 80 80 81 81 81 81
  line L56 (29.1627, -47.3434) -> (28.9185, -47.1664)
  spline S343 degree 3 poles (28.9185, -47.1664) (28.2477, -46.6789) (27.5649, -46.2201) (26.778, -45.7069) knots 82 82 82 82 83 83 83 83
  spline S344 degree 3 poles (26.778, -45.7069) (27.8995, -45.4358) (28.8347, -44.7577) (29.4478, -44.2026) knots 83 83 83 83 84 84 84 84
  spline S345 degree 3 poles (29.4478, -44.2026) (29.9129, -43.7817) (30.4677, -43.1549) (30.6284, -42.8854) knots 84 84 84 84 85 85 85 85
  line L57 (30.6284, -42.8854) -> (30.6334, -42.8895)
  spline S346 degree 3 poles (30.6334, -42.8895) (30.6376, -42.8846) (30.6414, -42.8792) (30.6455, -42.8741) knots 86 86 86 86 87 87 87 87
  spline S347 degree 3 poles (30.6455, -42.8741) (31.0979, -43.2586) (31.5482, -43.6733) (32.0247, -44.148) knots 87 87 87 87 88 88 88 88
  line L58 (32.0247, -44.148) -> (33.1141, -45.0862)
  spline S348 degree 3 poles (33.1141, -45.0862) (33.7263, -45.6137) (34.4379, -46.2247) (35.1594, -46.8226) knots 89 89 89 89 90 90 90 90
  arc A8 (35.1594, -46.8226) -> (35.1923, -46.8629) centre (35.3118, -46.7321) ccw
  spline S349 degree 3 poles (35.1923, -46.8629) (35.6521, -47.2822) (36.3564, -47.9765) (37.2857, -48.9264) (38.1914, -49.8521) (38.9893, -50.6928) (38.9947, -50.6983) knots 91 91 91 91 92 92 92 93 93 93 93
  spline S350 degree 3 poles (64.6851, -61.6042) (66.6712, -60.0252) (69.7423, -60.6603) (70.3724, -60.813) knots 0 0 0 0 1 1 1 1
  ellipse E47 centre (13.5082, -15.869) end of major axis (-42.262, 33.5321) minor radius 17.0835 (68.9587, -65.5917) -> (70.3724, -60.813) ccw
  spline S351 degree 3 poles (68.9587, -65.5917) (66.998, -67.3493) (63.619, -66.8671) (62.91, -66.7418) knots 2 2 2 2 3 3 3 3
  ellipse E48 centre (120.2091, -121.3276) end of major axis (175.9804, -180.8375) minor radius 18.0713 (64.6851, -61.6042) -> (62.91, -66.7418) ccw
  spline S352 degree 3 poles (72.1468, -71.9181) (73.9919, -75.0912) (72.6257, -79.0462) (72.3193, -79.8393) knots 0 0 0 0 1 1 1 1
  ellipse E49 centre (231.6421, -21.5333) end of major axis (63.1578, -73.2543) minor radius 32.5963 (63.26, -73.5583) -> (72.3193, -79.8393) ccw
  spline S353 degree 3 poles (63.26, -73.5583) (62.2487, -70.7958) (63.6771, -68.2365) (63.9839, -67.7363) knots 2 2 2 2 3 3 3 3
  ellipse E50 centre (-42.9216, -146.0207) end of major axis (-157.8285, -220.3863) minor radius 29.7458 (72.1468, -71.9181) -> (63.9839, -67.7363) ccw
  spline S354 degree 3 poles (58.8655, -70.1606) (60.5915, -71.1887) (61.1764, -72.9864) (61.2984, -73.433) knots 0 0 0 0 1 1 1 1
  ellipse E51 centre (71.9084, -1.876) end of major axis (57.2999, -74.8245) minor radius 15.2836 (56.9464, -74.7321) -> (61.2984, -73.433) ccw
  spline S355 degree 3 poles (56.9464, -74.7321) (54.5999, -73.9718) (53.4474, -70.6069) (53.2071, -69.8186) knots 2 2 2 2 3 3 3 3
  ellipse E52 centre (21.4323, -133.3674) end of major axis (-15.9892, -196.5812) minor radius 19.1168 (58.8655, -70.1606) -> (53.2071, -69.8186) ccw
  ellipse E53 centre (-1.2446, -48.2344) end of major axis (-56.6675, -14.8915) minor radius 17.9655 (51.0689, -84.0386) -> (54.6377, -80.5834) ccw
  spline S356 degree 3 poles (51.0689, -84.0386) (50.7561, -83.875) (49.3847, -83.0657) (49.0235, -81.3026) knots 1 1 1 1 2 2 2 2
  spline S357 degree 3 poles (49.0235, -81.3026) (48.5514, -78.9978) (49.9811, -75.9383) (53.1601, -72.4448) knots 2 2 2 2 3 3 3 3
  spline S358 degree 3 poles (53.1601, -72.4448) (53.683, -73.3873) (55.7215, -77.3825) (54.6377, -80.5834) knots 3 3 3 3 4 4 4 4
  spline S359 degree 3 poles (48.713, -72.5127) (46.6569, -73.9992) (43.6171, -73.2254) (42.995, -73.0439) knots 0 0 0 0 1 1 1 1
  ellipse E54 centre (97.8279, -120.5969) end of major axis (44.2906, -68.6419) minor radius 17.0951 (44.6252, -68.3348) -> (42.995, -73.0439) ccw
  spline S360 degree 3 poles (44.6252, -68.3348) (46.664, -66.6683) (50.0176, -67.3041) (50.7202, -67.4616) knots 2 2 2 2 3 3 3 3
  ellipse E55 centre (-4.2063, -10.1431) end of major axis (48.9701, -72.3103) minor radius 18.1014 (48.713, -72.5127) -> (50.7202, -67.4616) ccw
  spline S361 degree 3 poles (36.0259, -54.2727) (35.7995, -54.3025) (35.5989, -54.1799) (35.3658, -54.0382) knots 0 0 0 0 1 1 1 1
  spline S362 degree 3 poles (35.3658, -54.0382) (35.3141, -54.0068) (35.2624, -53.9753) (35.2101, -53.9455) knots 1 1 1 1 2 2 2 2
  spline S363 degree 3 poles (35.2101, -53.9455) (34.955, -53.7997) (34.7114, -53.6309) (34.4759, -53.4677) knots 2 2 2 2 3 3 3 3
  spline S364 degree 3 poles (34.4759, -53.4677) (34.1659, -53.2529) (33.8455, -53.0308) (33.4851, -52.8498) knots 3 3 3 3 4 4 4 4
  line L59 (33.4851, -52.8498) -> (33.3632, -52.7889)
  spline S365 degree 3 poles (33.3632, -52.7889) (33.2321, -52.7236) (33.1006, -52.6582) (32.9732, -52.5862) knots 5 5 5 5 6 6 6 6
  spline S366 degree 3 poles (32.9732, -52.5862) (32.973, -52.5862) (32.973, -52.5861) (32.973, -52.5861) knots 6 6 6 6 7 7 7 7
  spline S367 degree 3 poles (32.973, -52.5861) (32.9117, -52.5516) (32.8419, -52.5168) (32.7689, -52.4804) knots 7 7 7 7 8 8 8 8
  spline S368 degree 3 poles (32.7689, -52.4804) (32.7386, -52.4654) (32.7074, -52.4498) (32.6759, -52.4338) knots 8 8 8 8 9 9 9 9
  spline S369 degree 3 poles (32.6759, -52.4338) (32.4555, -52.3217) (32.2213, -52.1854) (32.1939, -52.0141) knots 9 9 9 9 10 10 10 10
  ellipse E56 centre (32.805, -51.9626) end of major axis (33.0158, -52.7055) minor radius 0.609 (32.1841, -51.8116) -> (32.1939, -52.0141) ccw
  spline S370 degree 3 poles (32.1841, -51.8116) (32.2254, -51.1528) (32.8087, -50.6185) (33.3234, -50.1472) knots 11 11 11 11 12 12 12 12
  spline S371 degree 3 poles (33.3234, -50.1472) (33.3949, -50.0817) (33.4646, -50.0177) (33.5309, -49.9553) knots 12 12 12 12 13 13 13 13
  spline S372 degree 3 poles (33.5309, -49.9553) (33.9907, -49.523) (34.6308, -49.0247) (35.5082, -49.0078) knots 13 13 13 13 14 14 14 14
  spline S373 degree 3 poles (35.5082, -49.0078) (35.6223, -49.004) (35.7024, -49.0436) (35.7539, -49.1241) knots 14 14 14 14 15 15 15 15
  spline S374 degree 3 poles (35.7539, -49.1241) (35.8283, -49.2405) (35.8195, -49.4039) (35.7737, -49.4983) knots 15 15 15 15 16 16 16 16
  spline S375 degree 3 poles (35.7737, -49.4983) (35.7017, -49.6459) (35.5678, -49.7644) (35.4263, -49.8899) knots 16 16 16 16 17 17 17 17
  spline S376 degree 3 poles (35.4263, -49.8899) (35.3355, -49.9704) (35.2414, -50.0536) (35.1589, -50.1492) (34.8761, -50.4769) (34.541, -50.927) (34.4597, -51.503) knots 17 17 17 17 18 18 18 19 19 19 19
  spline S377 degree 3 poles (34.4597, -51.503) (34.4451, -51.6074) (34.4006, -51.9254) (34.6094, -52.0465) knots 19 19 19 19 20 20 20 20
  spline S378 degree 3 poles (34.6094, -52.0465) (34.6527, -52.0716) (34.6997, -52.0842) (34.75, -52.0842) (34.849, -52.0842) (34.9615, -52.0358) (35.086, -51.9394) knots 20 20 20 20 21 21 21 22 22 22 22
  spline S379 degree 3 poles (35.086, -51.9394) (35.4698, -51.6422) (35.6836, -51.2324) (35.8905, -50.836) knots 22 22 22 22 23 23 23 23
  spline S380 degree 3 poles (35.8905, -50.836) (35.9261, -50.7676) (35.9618, -50.6994) (35.9981, -50.6319) knots 23 23 23 23 24 24 24 24
  spline S381 degree 3 poles (35.9981, -50.6319) (36.0197, -50.5919) (36.0417, -50.5496) (36.0645, -50.506) knots 24 24 24 24 25 25 25 25
  spline S382 degree 3 poles (36.0645, -50.506) (36.2183, -50.2104) (36.4097, -49.8424) (36.7123, -49.757) knots 25 25 25 25 26 26 26 26
  spline S383 degree 3 poles (36.7123, -49.757) (36.8852, -49.7083) (37.125, -49.7995) (37.1877, -49.995) knots 26 26 26 26 27 27 27 27
  ellipse E57 centre (36.4592, -50.9582) end of major axis (36.6476, -52.9758) minor radius 0.9074 (37.3807, -51.3993) -> (37.1877, -49.995) ccw
  spline S384 degree 3 poles (37.3807, -51.3993) (37.361, -52.1631) (37.1028, -53.0031) (36.6722, -53.7039) knots 28 28 28 28 29 29 29 29
  spline S385 degree 3 poles (36.6722, -53.7039) (36.5039, -53.9772) (36.3091, -54.2354) (36.0259, -54.2727) knots 29 29 29 29 30 30 30 30
  spline S386 degree 3 poles (17.161, -41.1673) (16.9263, -41.4298) (16.6636, -41.6702) (16.3492, -41.6555) knots 0 0 0 0 1 1 1 1
  spline S387 degree 3 poles (16.3492, -41.6555) (16.0969, -41.6434) (15.9034, -41.4723) (15.6793, -41.2742) knots 1 1 1 1 2 2 2 2
  spline S388 degree 3 poles (15.6793, -41.2742) (15.6302, -41.2307) (15.5808, -41.1871) (15.5305, -41.145) (15.2854, -40.9398) (15.0573, -40.7121) (14.8366, -40.4918) knots 2 2 2 2 3 3 3 4 4 4 4
  spline S389 degree 3 poles (14.8366, -40.4918) (14.5474, -40.2031) (14.2482, -39.9046) (13.8989, -39.6424) knots 4 4 4 4 5 5 5 5
  line L60 (13.8989, -39.6424) -> (13.7912, -39.5619)
  spline S390 degree 3 poles (13.7912, -39.5619) (13.6613, -39.4653) (13.5272, -39.3655) (13.4021, -39.2617) knots 6 6 6 6 7 7 7 7
  spline S391 degree 3 poles (13.4021, -39.2617) (13.4021, -39.2616) (13.4021, -39.2616) (13.4019, -39.2615) knots 7 7 7 7 8 8 8 8
  spline S392 degree 3 poles (13.4019, -39.2615) (13.3432, -39.2129) (13.2753, -39.1621) (13.2044, -39.1092) knots 8 8 8 8 9 9 9 9
  spline S393 degree 3 poles (13.2044, -39.1092) (12.9663, -38.9318) (12.6698, -38.711) (12.6742, -38.4877) knots 9 9 9 9 10 10 10 10
  ellipse E58 centre (13.1969, -38.3536) end of major axis (12.9858, -39.0558) minor radius 0.4995 (12.7031, -38.2667) -> (12.6742, -38.4877) ccw
  spline S394 degree 3 poles (12.7031, -38.2667) (12.8757, -37.5645) (13.6048, -37.1043) (14.248, -36.6981) knots 11 11 11 11 12 12 12 12
  spline S395 degree 3 poles (14.248, -36.6981) (14.3371, -36.6419) (14.4239, -36.5872) (14.5068, -36.5332) knots 12 12 12 12 13 13 13 13
  spline S396 degree 3 poles (14.5068, -36.5332) (15.0837, -36.1582) (15.8686, -35.7471) (16.8126, -35.8988) knots 13 13 13 13 14 14 14 14
  ellipse E59 centre (13.3209, -39.3795) end of major axis (9.6294, -42.7625) minor radius 1.1539 (17.0648, -36.0801) -> (16.8126, -35.8988) ccw
  spline S397 degree 3 poles (17.0648, -36.0801) (17.1166, -36.2062) (17.0939, -36.3859) (17.0117, -36.4982) knots 15 15 15 15 16 16 16 16
  spline S398 degree 3 poles (17.0117, -36.4982) (16.9049, -36.6445) (16.7375, -36.7463) (16.5604, -36.8543) knots 16 16 16 16 17 17 17 17
  spline S399 degree 3 poles (16.5604, -36.8543) (16.4484, -36.9224) (16.3325, -36.9928) (16.2267, -37.0784) knots 17 17 17 17 18 18 18 18
  spline S400 degree 3 poles (16.2267, -37.0784) (15.8629, -37.3733) (15.4201, -37.7882) (15.224, -38.3832) knots 18 18 18 18 19 19 19 19
  spline S401 degree 3 poles (15.224, -38.3832) (15.1288, -38.6731) (15.1455, -38.8673) (15.2747, -38.9769) knots 19 19 19 19 20 20 20 20
  spline S402 degree 3 poles (15.2747, -38.9769) (15.3357, -39.0287) (15.4056, -39.047) (15.4745, -39.047) (15.6059, -39.047) (15.7334, -38.9803) (15.7878, -38.9519) knots 20 20 20 20 21 21 21 22 22 22 22
  spline S403 degree 3 poles (15.7878, -38.9519) (16.2527, -38.7096) (16.5595, -38.3135) (16.8563, -37.9305) knots 22 22 22 22 23 23 23 23
  spline S404 degree 3 poles (16.8563, -37.9305) (16.9071, -37.8648) (16.958, -37.7992) (17.0095, -37.7346) knots 23 23 23 23 24 24 24 24